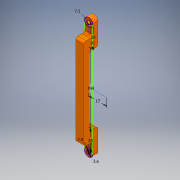
# Autodesk Inventor part: 防傾桿
Saved by Autodesk Inventor 2019 (Build 230136000, 136)
## iProperties
Created: 2020-03-19
Part Number: 防傾桿
Material: 一般
Document SubType Name: Modeling
Designer: 吳昇峻
Density: 1 g/cm^3
Appearance: 預設
Author: 吳昇峻
Autodesk Inventor part; units mm, degrees
ref_plane "YZ Plane" through (0, 0, 0) normal (1, 0, 0) x (0, 1, 0)
ref_plane "XZ Plane" through (0, 0, 0) normal (0, 1, 0) x (-1, 0, 0)
ref_plane "XY Plane" through (0, 0, 0) normal (0, 0, 1) x (1, 0, 0)
sketch "草圖1" plane through (0, 0, 0) normal (0, 1, 0) x (-1, 0, 0)
  circle A0 centre (0, 0) radius 1.8
  line L0 (0, 0) -> (0, -104) construction
  circle A1 centre (0, -104) radius 1.8
  line L1 (0, -52) -> (-17, -52) construction
  circle A2 centre (0, -104) radius 3.75
  circle A3 centre (0, 0) radius 3.75
  line L2 (-3.75, -104) -> (-3.75, 0)
  line L3 (3.75, -104) -> (3.75, 0)
  line L4 (0, 0) -> (0, -20) construction
  line L5 (0, -104) -> (0, -84) construction
  line L6 (3.75, -84) -> (-3.75, -84)
  line L7 (3.75, -20) -> (-3.75, -20)
  line L8 (0, -20) -> (0, -30) construction
  line L9 (0, -84) -> (0, -74) construction
  line L10 (0, -20) -> (0, -10) construction
  line L11 (0, -84) -> (0, -94) construction
  line L12 (3.75, -94) -> (-3.75, -94)
  line L13 (3.75, -10) -> (-3.75, -10)
  dimension "d0" = 3.6
  dimension "d1" = 104
  dimension "d2" = 3.6
  dimension "d7" = 17
  dimension "d18" = 7.5
  dimension "d19" = 7.5
  dimension "d25" = 20
  dimension "d26" = 20
  dimension "d29" = 10
  constraints: 28 end point, 12 point on line, 4 centre point, 4 coincident, 4 perpendicular, 4 point on circle, 3 midpoint, 2 tangent, 1 horizontal, 1 vertical
  measures "d0" diameter of A0
  measures "d1" distance of L0.start L0.end
  measures "d2" diameter of A1
  measures "d7" distance of L1.start L1.end
  measures "d18" diameter of A2
  measures "d19" diameter of A3
  measures "d25" distance of L4.start L4.end
  measures "d26" distance of L5.start L5.end
  measures "d29" distance of L4.end L10.end
extrude "Extrusion5" add sketch "草圖1" along normal blind 5 contours A2 | A2 L2 L12 L3 | L12 L2 L6 L3 | L7 L2 L13 L3 | L13 L2 A3 L3 | A3
fillet "Fillet4" radius 2 2 edges at (0, 5, -20) (0, 5, -84)
extrude "Extrusion7" add sketch "草圖1" against normal blind 3 contours L12 L2 L6 L3 | L7 L2 L13 L3
sketch "Sketch2" plane through (0, -3, 0) normal (0, -1, 0) x (1, 0, 0)
  line L0 (3.75, -104) -> (3.75, 0) projected
  line L1 (-3.75, -104) -> (-3.75, 0) projected
  line L2 (-3.75, -20) -> (3.75, -20) projected
  line L3 (3.75, -10) -> (-3.75, -10) projected
  line L4 (3.75, -84) -> (-3.75, -84) projected
  line L5 (-3.75, -94) -> (3.75, -94) projected
  point P0 (0, 0)
extrude "Extrusion8" add sketch "Sketch2" along normal blind 5
fillet "Fillet5" radius 2 6 edges at (0, -8, -94) (0, -8, -10) (0, 0, -10) (0, -3, -20) (0, -3, -84) (0, 0, -94)
body "Solid4"
